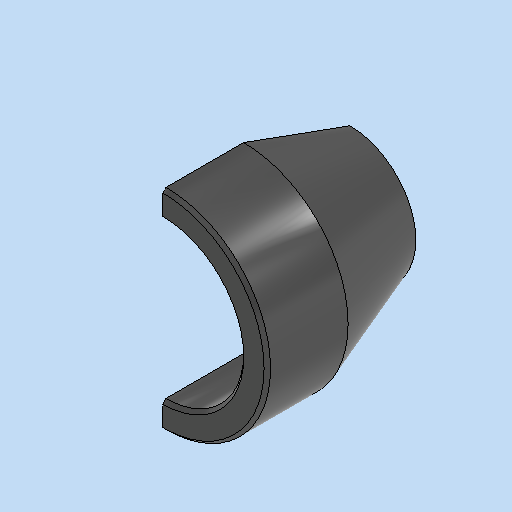
# Autodesk Inventor part: FujiiEchelleColilmatorAttachement
Saved by Autodesk Inventor 2025 (Build 290162000, 162)
## iProperties
Created: 2025-02-14
Part Number: FujiiEchelleColilmatorAttachement
Material: ABS Plastic
Document SubType Name: Modeling
Designer: kuzmin
Density: 1.06 g/cm^3
Appearance: Dark Gray
Author: kuzmin
Autodesk Inventor part; units mm, degrees
ref_plane "YZ Plane" through (0, 0, 0) normal (1, 0, 0) x (0, 1, 0)
ref_plane "XZ Plane" through (0, 0, 0) normal (0, 1, 0) x (-1, 0, 0)
ref_plane "XY Plane" through (0, 0, 0) normal (0, 0, 1) x (1, 0, 0)
sketch "Sketch1" plane through (0, 0, 0) normal (0, 0, 1) x (1, 0, 0)
  circle A0 centre (0, 0) radius 32.5
  dimension "d0" = 65
  constraints: 1 centre point, 1 coincident
  measures "d0" diameter of A0
extrude "Extrusion1" add sketch "Sketch1" along normal blind 58
sketch "Sketch2" plane through (0, 0, 58) normal (0, 0, 1) x (1, 0, 0)
  circle A0 centre (0, 0) radius 24.2
  dimension "d3" = 48.4
  constraints: 1 centre point, 1 coincident
  measures "d3" diameter of A0
extrude "Extrusion2" cut sketch "Sketch2" against normal blind 30
sketch "Sketch3" plane through (0, 0, 0) normal (0, 0, -1) x (-1, 0, 0)
  circle A0 centre (0, 0) radius 12.15
  dimension "d6" = 24.3
  constraints: 1 centre point, 1 coincident
  measures "d6" diameter of A0
extrude "Extrusion3" cut sketch "Sketch3" against normal through all
sketch "Sketch4" plane through (0, 0, 0) normal (0, 0, -1) x (-1, 0, 0)
  circle A0 centre (0, 0) radius 16 construction
  point P0 (-16, 0)
  point P1 (16, 0)
  point P2 (0, -16)
  point P3 (0, 16)
  dimension "d9" = 32
  constraints: 4 point on circle, 2 horizontal alignment, 2 vertical alignment, 1 centre point, 1 coincident
  measures "d9" diameter of A0
hole "Hole1" at (16, 0, 0) at (-16, 0, 0) at (0, -16, 0) at (0, 16, 0) direction (0, 0, 1) diameter 3 depth 10 tip angle 80
chamfer "Chamfer1" distance 1 angle 45 4 edges at (-32.5, 0, 58) (12.15, 0, 0) (-24.2, 0, 58) (12.15, 0, 28)
chamfer "Chamfer2" distance 0.4 angle 45 1 edges at (-24.2, 0, 28)
chamfer "Chamfer3" distance 12 angle 70 1 edges at (-32.5, 0, 0) measured on face at (9.1116, -18.0337, 0)
chamfer "Chamfer4" distance 0.4 angle 45 4 edges at (0, -17.5, 0) (-16, -1.5, 0) (16, -1.5, 0) (0, 14.5, 0)
body "Solid1"
